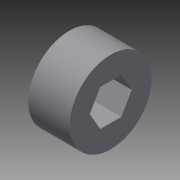
# Autodesk Inventor part: Spacer
Saved by Autodesk Inventor 2015 (Build 190159000, 159)
## iProperties
Created: 2015-02-14
Part Number: Spacer
Material: Generic
Document SubType Name: Modeling
Designer: whitaus15
Density: 1 g/cm^3
Appearance: Default
Author: whitaus15
Autodesk Inventor part; units mm, degrees
ref_plane "YZ Plane" through (0, 0, 0) normal (1, 0, 0) x (0, 1, 0)
ref_plane "XZ Plane" through (0, 0, 0) normal (0, 1, 0) x (-1, 0, 0)
ref_plane "XY Plane" through (0, 0, 0) normal (0, 0, 1) x (1, 0, 0)
sketch "Sketch1" plane through (0, 0, 0) normal (1, 0, 0) x (0, 1, 0)
  circle A0 centre (0, 0) radius 14.2875
  line L0 (0, -7.3323) -> (-6.35, -3.6662)
  line L1 (-6.35, -3.6662) -> (-6.35, 3.6662)
  line L2 (-6.35, 3.6662) -> (0, 7.3323)
  line L3 (0, 7.3323) -> (6.35, 3.6662)
  line L4 (6.35, 3.6662) -> (6.35, -3.6662)
  line L5 (6.35, -3.6662) -> (0, -7.3323)
  dimension "d1" = 28.575
  dimension "d4" = 12.7
  constraints: 12 end point, 1 centre point, 1 coincident, 13 other
  measures "d1" diameter of A0
  measures "d4" distance between parallel lines of L2 L5
extrude "Extrusion2" add sketch "Sketch1" along normal blind 14.478
body "Solid2"
